Autodesk Inventor part; units mm, degrees
(part 2 of 2)
sketch "Skizze29" plane through (89.6, -2.4765, -33.8) normal (0, 0, -1) x (-1, 0, 0)
  line L0 (43.6, -0.4235) -> (43.6, -0.5235) construction
  line L1 (43.6, -0.5235) -> (49.9, -0.5235) construction
  line L2 (49.9, -0.5235) -> (52.9, 2.4765) construction
  line L3 (52.9, 2.4765) -> (79.4, 2.4765) construction
  line L4 (79.4, 2.4765) -> (79.4, 2.2765) construction
  line L5 (79.4, 2.2765) -> (83.4, 2.2765) construction
  line L6 (83.4, 2.2765) -> (83.4, 7.3765) construction
  line L7 (83.4, 7.3765) -> (49.9, 7.3765) construction
  line L8 (49.9, 7.3765) -> (49.9, 6.7966) construction
  line L9 (49.9, 6.7966) -> (45.4981, 2.3946) construction
  line L10 (45.4981, 2.3946) -> (38.1019, 2.3946) construction
  line L11 (38.1019, 2.3946) -> (33.7, 6.7966) construction
  line L12 (33.7, 6.7966) -> (33.7, 7.3765) construction
  line L13 (33.7, 7.3765) -> (17.2925, 7.3765) construction
  line L14 (17.2925, 7.3765) -> (17.2925, 2.4765) construction
  line L15 (17.2925, 2.4765) -> (31.9, 2.4765) construction
  line L16 (31.9, 2.4765) -> (34.8, -0.4235) construction
  line L17 (34.8, -0.4235) -> (43.6, -0.4235) construction
  line L18 (43.6, -28.4235) -> (34.8, -28.4235) construction
  line L19 (31.9, -31.3235) -> (34.8, -28.4235) construction
  line L20 (17.2925, -31.3235) -> (31.9, -31.3235) construction
  line L21 (17.2925, -31.3235) -> (17.2925, -36.2235) construction
  line L22 (33.7, -36.2235) -> (17.2925, -36.2235) construction
  line L23 (33.7, -36.2235) -> (33.7, -35.6437) construction
  line L24 (38.1019, -31.2417) -> (33.7, -35.6437) construction
  line L25 (45.4981, -31.2417) -> (38.1019, -31.2417) construction
  line L26 (49.9, -35.6437) -> (45.4981, -31.2417) construction
  line L27 (49.9, -35.6437) -> (49.9, -36.2235) construction
  line L28 (83.4, -36.2235) -> (49.9, -36.2235) construction
  line L29 (83.4, -31.1235) -> (83.4, -36.2235) construction
  line L30 (83.4, -31.1235) -> (79.4, -31.1235) construction
  line L31 (79.4, -31.3235) -> (79.4, -31.1235) construction
  line L32 (52.9, -31.3235) -> (79.4, -31.3235) construction
  line L33 (49.9, -28.3235) -> (52.9, -31.3235) construction
  line L34 (43.6, -28.3235) -> (49.9, -28.3235) construction
  line L35 (43.6, -28.3235) -> (43.6, -28.4235) construction
  line L36 (6, -28.8471) -> (0, -28.8471) construction
  line L37 (0, -28.8471) -> (0, -36.2235) construction
  line L38 (0, -36.2235) -> (6, -36.2235) construction
  line L39 (6, -36.2235) -> (6, -28.8471) construction
  line L40 (0, 7.3765) -> (0, 0) construction
  line L41 (0, 0) -> (6, 0) construction
  line L42 (6, 0) -> (6, 7.3765) construction
  line L43 (6, 7.3765) -> (0, 7.3765) construction
  line L44 (0, -28.8471) -> (3.8, -28.8471) construction
  line L45 (3.8, -27.1235) -> (3.8, -28.8471) construction
  line L46 (-4.5838, -27.1235) -> (3.8, -27.1235) construction
  line L47 (-4.5838, -1.7235) -> (-4.5838, -27.1235) construction
  line L48 (-4.5838, -1.7235) -> (3.8, -1.7235) construction
  line L49 (3.8, -1.7235) -> (3.8, 0) construction
  line L50 (3.8, 0) -> (0, 0) construction
  line L51 (0, 0) -> (0, 2.2765) construction
  line L52 (0, 2.2765) -> (-8.2, 2.2765) construction
  line L53 (-8.2, 2.2765) -> (-8.2, -31.1235) construction
  line L54 (0, -31.1235) -> (-8.2, -31.1235) construction
  line L55 (0, -31.1235) -> (0, -28.8471) construction
  line L56 (17.2925, 7.3765) -> (-8.2, 7.3765)
  line L57 (-8.2, 7.3765) -> (-8.2, -36.2235)
  line L58 (-8.2, -36.2235) -> (17.2925, -36.2235)
  line L59 (17.2925, -36.2235) -> (17.2925, 7.3765)
  line L60 (0, -36.2235) -> (6, -36.2235) projected
  point P0 (89.6, 2.4765)
  point P1 (3.8, 2.4765)
  constraints: 8 end point, 2 collinear, 2 parallel, 1 horizontal, 1 perpendicular
extrude "Extrusion29" cut sketch "Skizze29" against normal through all
sketch "Skizze30" plane through (0, 0, 0) normal (0, 0, 1) x (1, 0, 0)
  line L0 (72.3075, -38.7) -> (72.3075, -33.8) construction
  line L1 (57.7, -33.8) -> (72.3075, -33.8) construction
  line L2 (57.7, -33.8) -> (54.8, -30.9) construction
  line L3 (54.8, -30.9) -> (42, -30.9) construction
  line L4 (42, -30.9) -> (42, -30.8) construction
  line L5 (42, -30.8) -> (39.7, -30.8) construction
  line L6 (39.7, -30.8) -> (36.7, -33.8) construction
  line L7 (10.2, -33.8) -> (36.7, -33.8) construction
  line L8 (10.2, -29.4029) -> (10.2, -33.8) construction
  arc A0 (10.2, -4.3971) -> (10.2, -29.4029) centre (14.0958, -16.9) ccw construction
  line L9 (10.2, -4.3971) -> (10.2, 0) construction
  line L10 (10.2, 0) -> (36.7, 0) construction
  line L11 (39.7, -3) -> (36.7, 0) construction
  line L12 (42, -3) -> (39.7, -3) construction
  line L13 (42, -3) -> (42, -2.9) construction
  line L14 (42, -2.9) -> (54.8, -2.9) construction
  line L15 (57.7, 0) -> (54.8, -2.9) construction
  line L16 (57.7, 0) -> (72.3075, 0) construction
  line L17 (72.3075, 0) -> (72.3075, 4.9) construction
  line L18 (72.3075, 4.9) -> (55.9, 4.9) construction
  line L19 (55.9, 4.9) -> (55.9, 4.3201) construction
  line L20 (51.4981, -0.0818) -> (55.9, 4.3201) construction
  line L21 (44.1019, -0.0818) -> (51.4981, -0.0818) construction
  line L22 (39.7, 4.3201) -> (44.1019, -0.0818) construction
  line L23 (39.7, 4.3201) -> (39.7, 4.9) construction
  line L24 (39.7, 4.9) -> (6.2, 4.9) construction
  line L25 (6.2, 4.9) -> (6.2, -0.2) construction
  line L26 (6.2, -0.2) -> (-2, -0.2) construction
  line L27 (-2, -0.2) -> (-2, -33.6) construction
  line L28 (6.2, -33.6) -> (-2, -33.6) construction
  line L29 (6.2, -38.7) -> (6.2, -33.6) construction
  line L30 (39.7, -38.7) -> (6.2, -38.7) construction
  line L31 (39.7, -38.7) -> (39.7, -38.1201) construction
  line L32 (39.7, -38.1201) -> (44.1019, -33.7182) construction
  line L33 (44.1019, -33.7182) -> (51.4981, -33.7182) construction
  line L34 (51.4981, -33.7182) -> (55.9, -38.1201) construction
  line L35 (55.9, -38.1201) -> (55.9, -38.7) construction
  line L36 (72.3075, -38.7) -> (55.9, -38.7) construction
  circle A1 centre (59.1, -36.25) radius 1.4
  line L37 (-16.8615, -16.9) -> (87.169, -16.9) construction
  circle A2 centre (59.1, 2.45) radius 1.4
  line L38 (72.3075, -38.7) -> (72.3075, -33.8) construction
  line L39 (72.3075, -36.25) -> (54.0299, -36.25) construction
  line L40 (51.4981, -33.7182) -> (55.9, -38.1201) construction
  line L41 (57.7, -33.8) -> (54.8, -30.9) construction
  line L42 (57.7, -33.8) -> (57.7, -38.7) construction
  point P0 (0, 0)
  dimension "d149" = 2.8
  constraints: 4 end point, 3 point on line, 2 centre point, 1 horizontal, 1 midpoint, 1 symmetric about line, 1 tangent, 1 vertical, 1 other
  measures "d149" diameter of A1
extrude "Extrusion30" cut sketch "Skizze30" against normal through all
fillet "Rundung1" radius 3 2 edges at (72.3075, -38.7, -3) (72.3075, 4.9, -3)
sketch "Skizze31" plane through (0, 0, 0) normal (0, 0, 1) x (1, 0, 0)
  circle A0 centre (59.1, -36.25) radius 1.4 construction
  circle A1 centre (59.1, 2.45) radius 1.4 construction
  arc A2 (72.3075, 1.9) -> (69.3075, 4.9) centre (69.3075, 1.9) ccw construction
  line L0 (69.3075, 4.9) -> (55.9, 4.9) construction
  line L1 (55.9, 4.9) -> (55.9, 4.3201) construction
  line L2 (51.4981, -0.0818) -> (55.9, 4.3201) construction
  line L3 (44.1019, -0.0818) -> (51.4981, -0.0818) construction
  line L4 (39.7, 4.3201) -> (44.1019, -0.0818) construction
  line L5 (39.7, 4.3201) -> (39.7, 4.9) construction
  line L6 (39.7, 4.9) -> (6.2, 4.9) construction
  line L7 (6.2, 4.9) -> (6.2, -0.2) construction
  line L8 (6.2, -0.2) -> (-2, -0.2) construction
  line L9 (-2, -0.2) -> (-2, -33.6) construction
  line L10 (6.2, -33.6) -> (-2, -33.6) construction
  line L11 (6.2, -38.7) -> (6.2, -33.6) construction
  line L12 (39.7, -38.7) -> (6.2, -38.7) construction
  line L13 (39.7, -38.7) -> (39.7, -38.1201) construction
  line L14 (39.7, -38.1201) -> (44.1019, -33.7182) construction
  line L15 (44.1019, -33.7182) -> (51.4981, -33.7182) construction
  line L16 (51.4981, -33.7182) -> (55.9, -38.1201) construction
  line L17 (55.9, -38.1201) -> (55.9, -38.7) construction
  line L18 (69.3075, -38.7) -> (55.9, -38.7) construction
  arc A3 (69.3075, -38.7) -> (72.3075, -35.7) centre (69.3075, -35.7) ccw construction
  line L19 (72.3075, -35.7) -> (72.3075, -33.8) construction
  line L20 (57.7, -33.8) -> (72.3075, -33.8) construction
  line L21 (57.7, -33.8) -> (54.8, -30.9) construction
  line L22 (54.8, -30.9) -> (42, -30.9) construction
  line L23 (42, -30.9) -> (42, -30.8) construction
  line L24 (42, -30.8) -> (39.7, -30.8) construction
  line L25 (39.7, -30.8) -> (36.7, -33.8) construction
  line L26 (10.2, -33.8) -> (36.7, -33.8) construction
  line L27 (10.2, -29.4029) -> (10.2, -33.8) construction
  arc A4 (10.2, -4.3971) -> (10.2, -29.4029) centre (14.0958, -16.9) ccw construction
  line L28 (10.2, -4.3971) -> (10.2, 0) construction
  line L29 (10.2, 0) -> (36.7, 0) construction
  line L30 (39.7, -3) -> (36.7, 0) construction
  line L31 (42, -3) -> (39.7, -3) construction
  line L32 (42, -3) -> (42, -2.9) construction
  line L33 (42, -2.9) -> (54.8, -2.9) construction
  line L34 (57.7, 0) -> (54.8, -2.9) construction
  line L35 (57.7, 0) -> (72.3075, 0) construction
  line L36 (72.3075, 0) -> (72.3075, 1.9) construction
  line L37 (6.2, 4.9) -> (39.8, 4.9)
  line L38 (39.8, 4.9) -> (39.8, 8)
  line L39 (39.8, 8) -> (6.2, 8)
  line L40 (6.2, 8) -> (6.2, 4.9)
  line L41 (-16.9858, -16.9) -> (87.9146, -16.9) projected
  line L42 (39.7, -38.1201) -> (39.7, -38.7) construction
  line L43 (39.7, -38.7) -> (6.2, -38.7) construction
  line L44 (6.2, -38.7) -> (39.8, -38.7)
  line L45 (39.8, -38.7) -> (39.8, -41.8)
  line L46 (39.8, -41.8) -> (6.2, -41.8)
  line L47 (6.2, -41.8) -> (6.2, -38.7)
  point P0 (0, 0)
  dimension "d153" = 33.6
  dimension "d154" = 49.8
  constraints: 20 end point, 3 symmetric about line, 2 parallel, 1 horizontal, 1 perpendicular
  measures "d153" distance of L38.end L39.end
  measures "d154" distance between parallel lines of L46 L39
extrude "Extrusion31" add sketch "Skizze31" against normal up to surface (6 mm away)
sketch "Sketch32" plane through (0, 0, -6) normal (0, 0, -1) x (-1, 0, 0)
  circle A0 centre (-59.1, -36.25) radius 1.4 projected
  circle A1 centre (-59.1, 2.45) radius 1.4 projected
  arc A2 (-69.3075, 4.9) -> (-72.3075, 1.9) centre (-69.3075, 1.9) ccw projected
  line L0 (-69.3075, 4.9) -> (-55.9, 4.9) projected
  line L1 (-55.9, 4.9) -> (-55.9, 4.3201) projected
  line L2 (-51.4981, -0.0818) -> (-55.9, 4.3201) projected
  line L3 (-44.1019, -0.0818) -> (-51.4981, -0.0818) projected
  line L4 (-39.7, 4.3201) -> (-44.1019, -0.0818) projected
  line L5 (-39.7, 4.3201) -> (-39.7, 4.9) projected
  line L6 (-39.7, 4.9) -> (-39.8, 4.9) projected
  line L7 (-39.8, 4.9) -> (-39.8, 8) projected
  line L8 (-39.8, 8) -> (-6.2, 8) projected
  line L9 (-6.2, 8) -> (-6.2, -0.2) projected
  line L10 (-6.2, -0.2) -> (2, -0.2) projected
  line L11 (2, -0.2) -> (2, -33.6) projected
  line L12 (-6.2, -33.6) -> (2, -33.6) projected
  line L13 (-6.2, -41.8) -> (-6.2, -33.6) projected
  line L14 (-39.8, -41.8) -> (-6.2, -41.8) projected
  line L15 (-39.8, -38.7) -> (-39.8, -41.8) projected
  line L16 (-39.7, -38.7) -> (-39.8, -38.7) projected
  line L17 (-39.7, -38.7) -> (-39.7, -38.1201) projected
  line L18 (-39.7, -38.1201) -> (-44.1019, -33.7182) projected
  line L19 (-44.1019, -33.7182) -> (-51.4981, -33.7182) projected
  line L20 (-51.4981, -33.7182) -> (-55.9, -38.1201) projected
  line L21 (-55.9, -38.1201) -> (-55.9, -38.7) projected
  line L22 (-69.3075, -38.7) -> (-55.9, -38.7) projected
  arc A3 (-72.3075, -35.7) -> (-69.3075, -38.7) centre (-69.3075, -35.7) ccw projected
  line L23 (-72.3075, -35.7) -> (-72.3075, -33.8) projected
  line L24 (-57.7, -33.8) -> (-72.3075, -33.8) projected
  line L25 (-57.7, -33.8) -> (-54.8, -30.9) projected
  line L26 (-54.8, -30.9) -> (-42, -30.9) projected
  line L27 (-42, -30.9) -> (-42, -30.8) projected
  line L28 (-42, -30.8) -> (-39.7, -30.8) projected
  line L29 (-39.7, -30.8) -> (-36.7, -33.8) projected
  line L30 (-10.2, -33.8) -> (-36.7, -33.8) projected
  line L31 (-10.2, -29.4029) -> (-10.2, -33.8) projected
  arc A4 (-10.2, -29.4029) -> (-10.2, -4.3971) centre (-14.0958, -16.9) ccw projected
  line L32 (-10.2, -4.3971) -> (-10.2, 0) projected
  line L33 (-10.2, 0) -> (-36.7, 0) projected
  line L34 (-39.7, -3) -> (-36.7, 0) projected
  line L35 (-42, -3) -> (-39.7, -3) projected
  line L36 (-42, -3) -> (-42, -2.9) projected
  line L37 (-42, -2.9) -> (-54.8, -2.9) projected
  line L38 (-57.7, 0) -> (-54.8, -2.9) projected
  line L39 (-57.7, 0) -> (-72.3075, 0) projected
  line L40 (-72.3075, 0) -> (-72.3075, 1.9) projected
  line L41 (-48.0005, -33.7182) -> (-48.0005, -30.9)
  line L42 (-54.8, -30.9) -> (-42, -30.9) projected
  line L43 (-54.8, -2.9) -> (-46, -2.9) projected
  line L44 (-48.0005, -2.9) -> (-48.0005, -0.0818)
  line L45 (-44.1019, -0.0818) -> (-51.4981, -0.0818) projected
  point P0 (0, 0)
  dimension "d157" = 24.307
  constraints: 6 point on line, 4 end point, 1 perpendicular
  measures "d157" distance between parallel lines of L23 L41
extrude "Extrusion32" add sketch "Sketch32" along normal blind 7 contours A0 | A1 | L0 L1 L2 L3 L44 L37 L38 L39 L40 A2 | L41 L19 L20 L21 L22 A3 L23 L24 L25 L26
sketch "Sketch33" plane through (0, 0, 0) normal (0, 0, 1) x (1, 0, 0)
  circle A0 centre (59.1, -36.25) radius 1.4 projected
  circle A1 centre (59.1, 2.45) radius 1.4 projected
  arc A2 (72.3075, 1.9) -> (69.3075, 4.9) centre (69.3075, 1.9) ccw projected
  line L0 (69.3075, 4.9) -> (55.9, 4.9) projected
  line L1 (55.9, 4.9) -> (55.9, 4.3201) projected
  line L2 (51.4981, -0.0818) -> (55.9, 4.3201) projected
  line L3 (44.1019, -0.0818) -> (51.4981, -0.0818) projected
  line L4 (39.7, 4.3201) -> (44.1019, -0.0818) projected
  line L5 (39.7, 4.3201) -> (39.7, 4.9) projected
  line L6 (39.7, 4.9) -> (39.8, 4.9) projected
  line L7 (39.8, 4.9) -> (39.8, 8) projected
  line L8 (39.8, 8) -> (6.2, 8) projected
  line L9 (6.2, 8) -> (6.2, -0.2) projected
  line L10 (6.2, -0.2) -> (-2, -0.2) projected
  line L11 (-2, -0.2) -> (-2, -33.6) projected
  line L12 (6.2, -33.6) -> (-2, -33.6) projected
  line L13 (6.2, -41.8) -> (6.2, -33.6) projected
  line L14 (39.8, -41.8) -> (6.2, -41.8) projected
  line L15 (39.8, -38.7) -> (39.8, -41.8) projected
  line L16 (39.7, -38.7) -> (39.8, -38.7) projected
  line L17 (39.7, -38.7) -> (39.7, -38.1201) projected
  line L18 (39.7, -38.1201) -> (44.1019, -33.7182) projected
  line L19 (44.1019, -33.7182) -> (51.4981, -33.7182) projected
  line L20 (51.4981, -33.7182) -> (55.9, -38.1201) projected
  line L21 (55.9, -38.1201) -> (55.9, -38.7) projected
  line L22 (69.3075, -38.7) -> (55.9, -38.7) projected
  arc A3 (69.3075, -38.7) -> (72.3075, -35.7) centre (69.3075, -35.7) ccw projected
  line L23 (72.3075, -35.7) -> (72.3075, -33.8) projected
  line L24 (57.7, -33.8) -> (72.3075, -33.8) projected
  line L25 (57.7, -33.8) -> (54.8, -30.9) projected
  line L26 (54.8, -30.9) -> (42, -30.9) projected
  line L27 (42, -30.9) -> (42, -30.8) projected
  line L28 (42, -30.8) -> (39.7, -30.8) projected
  line L29 (39.7, -30.8) -> (36.7, -33.8) projected
  line L30 (10.2, -33.8) -> (36.7, -33.8) projected
  line L31 (10.2, -29.4029) -> (10.2, -33.8) projected
  arc A4 (10.2, -4.3971) -> (10.2, -29.4029) centre (14.0958, -16.9) ccw projected
  line L32 (10.2, -4.3971) -> (10.2, 0) projected
  line L33 (10.2, 0) -> (36.7, 0) projected
  line L34 (39.7, -3) -> (36.7, 0) projected
  line L35 (42, -3) -> (39.7, -3) projected
  line L36 (42, -3) -> (42, -2.9) projected
  line L37 (42, -2.9) -> (54.8, -2.9) projected
  line L38 (57.7, 0) -> (54.8, -2.9) projected
  line L39 (57.7, 0) -> (72.3075, 0) projected
  line L40 (72.3075, 0) -> (72.3075, 1.9) projected
  line L41 (69.3075, 4.9) -> (55.9, 4.9) projected
  line L42 (55.9, 4.9) -> (48.0005, 4.9)
  line L43 (48.0005, 4.9) -> (48.0005, -0.0818)
  line L44 (44.1019, -33.7182) -> (51.4981, -33.7182) projected
  line L45 (48.0005, -33.7182) -> (48.0005, -38.7)
  line L46 (48.0005, -38.7) -> (55.9, -38.7)
  point P0 (0, 0)
  dimension "d160" = 24.307
  constraints: 8 end point, 4 point on line, 2 perpendicular, 1 horizontal
  measures "d160" distance between parallel lines of L40 L43
extrude "Extrusion33" add sketch "Sketch33" against normal up to surface (13 mm away) contours A0 | A1 | L1 L2 L3 L43 L42 | L19 L20 L21 L46 L45
sketch "Sketch34" plane through (0, 0, -13) normal (0, 0, -1) x (-1, 0, 0)
  line L0 (-48.0005, -38.7) -> (-48.0005, -30.9) projected
  line L1 (-48.0005, -30.9) -> (-54.8, -30.9) projected
  line L2 (-54.8, -30.9) -> (-57.7, -33.8) projected
  line L3 (-57.7, -33.8) -> (-72.3075, -33.8) projected
  line L4 (-72.3075, -33.8) -> (-72.3075, -35.7) projected
  arc A0 (-72.3075, -35.7) -> (-69.3075, -38.7) centre (-69.3075, -35.7) ccw projected
  line L5 (-69.3075, -38.7) -> (-48.0005, -38.7) projected
  line L6 (-72.3075, 1.9) -> (-72.3075, 0) projected
  line L7 (-72.3075, 0) -> (-57.7, 0) projected
  line L8 (-57.7, 0) -> (-54.8, -2.9) projected
  line L9 (-54.8, -2.9) -> (-48.0005, -2.9) projected
  line L10 (-48.0005, -2.9) -> (-48.0005, 4.9) projected
  line L11 (-48.0005, 4.9) -> (-69.3075, 4.9) projected
  arc A1 (-69.3075, 4.9) -> (-72.3075, 1.9) centre (-69.3075, 1.9) ccw projected
  line L12 (-48.0005, -0.0818) -> (-48.0005, -2.9) projected
  line L13 (-48.0005, -30.9) -> (-48.0005, -2.9)
  line L14 (-72.3075, -33.8) -> (-72.3075, 0)
  point P0 (0, 0)
  constraints: 4 end point, 2 vertical
extrude "Extrusion34" add sketch "Sketch34" along normal blind 1
sketch "Sketch35" plane through (0, 0, -14) normal (0, 0, -1) x (-1, 0, 0)
  line L0 (-48.0005, -38.7) -> (-48.0005, 4.9) projected
  line L1 (-48.0005, 4.9) -> (-69.3075, 4.9) projected
  arc A0 (-69.3075, 4.9) -> (-72.3075, 1.9) centre (-69.3075, 1.9) ccw projected
  line L2 (-72.3075, 1.9) -> (-72.3075, -35.7) projected
  arc A1 (-72.3075, -35.7) -> (-69.3075, -38.7) centre (-69.3075, -35.7) ccw projected
  line L3 (-69.3075, -38.7) -> (-48.0005, -38.7) projected
  line L4 (-87.9146, -16.9) -> (16.9858, -16.9) construction
  line L5 (-48.0005, -33.8) -> (-72.3075, -33.8)
  line L6 (-72.3075, 1.9) -> (-72.3075, -35.7) construction
  line L7 (-48.0005, 0) -> (-72.3075, 0)
  line L8 (-48.0005, -33.7182) -> (-48.0005, -38.7) projected
  line L9 (-48.0005, -33.8) -> (-48.0005, -38.7)
  line L10 (-48.0005, -38.7) -> (-69.3075, -38.7)
  arc A2 (-72.3075, -35.7) -> (-69.3075, -38.7) centre (-69.3075, -35.7) ccw projected
  line L11 (-72.3075, -33.8) -> (-72.3075, -35.7)
  line L12 (-48.0005, 4.9) -> (-48.0005, -0.0818) projected
  line L13 (-48.0005, 0) -> (-48.0005, 4.9)
  line L14 (-48.0005, 4.9) -> (-69.3075, 4.9)
  line L15 (-69.263, 4.9) -> (-66.363, 4.9) projected
  line L16 (-72.3075, 0) -> (-72.3075, 1.9) projected
  line L17 (-72.3075, 0) -> (-72.3075, 1.9)
  arc A3 (-69.3075, 4.9) -> (-72.3075, 1.9) centre (-69.3075, 1.9) ccw projected
  arc A4 (-69.3075, 4.9) -> (-72.3075, 1.9) centre (-69.3075, 1.9) ccw
  arc A5 (-72.3075, -35.7) -> (-69.3075, -38.7) centre (-69.3075, -35.7) ccw
  point P0 (0, 0)
  dimension "d165" = 4.9
  constraints: 16 end point, 4 collinear, 4 point on circle, 2 centre point, 2 concentric, 2 perpendicular, 2 point on line, 2 symmetric about line, 2 tangent, 1 vertical
  measures "d165" distance between parallel lines of L3 L5
extrude "Extrusion35" add sketch "Sketch35" along normal blind 5.5 contours L3 A1 L2 L5 L0 | L2 A0 L1 L0 L7
sketch "Sketch36" plane through (0, 0, -19.5) normal (0, 0, -1) x (-1, 0, 0)
  line L0 (-48.0005, -38.7) -> (-48.0005, -33.8) projected
  line L1 (-48.0005, -33.8) -> (-72.3075, -33.8) projected
  line L2 (-72.3075, -33.8) -> (-72.3075, -35.7) projected
  arc A0 (-72.3075, -35.7) -> (-69.3075, -38.7) centre (-69.3075, -35.7) ccw projected
  line L3 (-69.3075, -38.7) -> (-48.0005, -38.7) projected
  line L4 (-72.3075, -33.8) -> (-48.0005, -33.8) projected
  line L5 (-48.0005, -33.8) -> (-48.0005, 0) projected
  line L6 (-48.0005, 0) -> (-72.3075, 0) projected
  line L7 (-72.3075, 0) -> (-72.3075, -33.8) projected
  line L8 (-48.0005, 4.9) -> (-69.3075, 4.9) projected
  arc A1 (-69.3075, 4.9) -> (-72.3075, 1.9) centre (-69.3075, 1.9) ccw projected
  line L9 (-72.3075, 1.9) -> (-72.3075, 0) projected
  line L10 (-72.3075, 0) -> (-48.0005, 0) projected
  line L11 (-48.0005, 0) -> (-48.0005, 4.9) projected
  point P0 (0, 0)
extrude "Extrusion36" add sketch "Sketch36" along normal blind 2
sketch "Sketch37" plane through (0, 0, -21.5) normal (0, 0, -1) x (-1, 0, 0)
  line L0 (-61, -23.9) -> (-71, -23.9) construction
  line L1 (-48.0005, -38.7) -> (-48.0005, 4.9) construction
  line L2 (-48.0005, 4.9) -> (-69.3075, 4.9) construction
  arc A0 (-69.3075, 4.9) -> (-72.3075, 1.9) centre (-69.3075, 1.9) ccw construction
  line L3 (-72.3075, 1.9) -> (-72.3075, -35.7) construction
  arc A1 (-72.3075, -35.7) -> (-69.3075, -38.7) centre (-69.3075, -35.7) ccw construction
  line L4 (-69.3075, -38.7) -> (-48.0005, -38.7) construction
  line L5 (-87.9146, -16.9) -> (16.9858, -16.9) construction
  circle A2 centre (-67.2465, -16.9) radius 1.7
  point P0 (0, 0)
  dimension "d170" = 5.061
  dimension "d171" = 3.4
  constraints: 1 centre point, 1 point on line
  measures "d170" distance from line of L3 A2.centre
  measures "d171" diameter of A2
extrude "Extrusion37" cut sketch "Sketch37" against normal up to surface (8.5 mm away)
sketch "Sketch38" plane through (0, 0, -13) normal (0, 0, 1) x (1, 0, 0)
  circle A0 centre (67.2465, -16.9) radius 1.7 construction
  line L0 (54.8, -2.9) -> (48.0005, -2.9) construction
  line L1 (48.0005, -30.9) -> (48.0005, -2.9) construction
  line L2 (48.0005, -30.9) -> (54.8, -30.9) construction
  line L3 (54.8, -30.9) -> (57.7, -33.8) construction
  line L4 (57.7, -33.8) -> (72.3075, -33.8) construction
  line L5 (72.3075, 0) -> (72.3075, -33.8) construction
  line L6 (72.3075, 0) -> (57.7, 0) construction
  line L7 (57.7, 0) -> (54.8, -2.9) construction
  circle A1 centre (67.2465, -16.9) radius 2.3
  point P0 (0, 0)
  dimension "d174" = 0.6
  constraints: 1 centre point
  measures "d174" radial gap between concentric circles of A0 A1
extrude "Extrusion38" cut sketch "Sketch38" against normal up to surface (1 mm away)
sketch "Sketch39" plane through (0, 0, -21.5) normal (0, 0, -1) x (-1, 0, 0)
  circle A0 centre (-67.2465, -16.9) radius 1.7 construction
  line L0 (-48.0005, -38.7) -> (-48.0005, 4.9) construction
  line L1 (-48.0005, 4.9) -> (-69.3075, 4.9) construction
  arc A1 (-69.3075, 4.9) -> (-72.3075, 1.9) centre (-69.3075, 1.9) ccw construction
  line L2 (-72.3075, 1.9) -> (-72.3075, -35.7) construction
  arc A2 (-72.3075, -35.7) -> (-69.3075, -38.7) centre (-69.3075, -35.7) ccw construction
  line L3 (-69.3075, -38.7) -> (-48.0005, -38.7) construction
  line L4 (-49.7605, -33.742) -> (-54.8216, -33.742) construction
  line L5 (-54.8216, -33.742) -> (-54.8216, -27.0483) construction
  line L6 (-54.8216, -27.0483) -> (-49.7605, -27.0483) construction
  line L7 (-49.7605, -27.0483) -> (-49.7605, -33.742) construction
  line L8 (-49.7605, -4.0192) -> (-54.9849, -4.0192) construction
  line L9 (-54.9849, -4.0192) -> (-54.9849, 2.6745) construction
  line L10 (-54.9849, 2.6745) -> (-49.7605, 2.6745) construction
  line L11 (-49.7605, 2.6745) -> (-49.7605, -4.0192) construction
  line L12 (-50.1879, -33.6727) -> (-52.0242, -33.6727)
  spline S0 degree 2 poles (-52.0242, -33.6727) (-52.5671, -33.6727) (-53.2369, -33.3763) (-53.672, -32.8258) (-53.8683, -32.0943) (-53.8683, -31.6862) knots 0 0 0 1 2 3 4 4 4
  spline S1 degree 2 poles (-53.8683, -31.6862) (-53.8683, -31.0433) (-53.5757, -30.3388) (-53.0598, -29.8614) (-52.7596, -29.7805) knots 0 0 0 1 2 3 3 3
  spline S2 degree 2 poles (-52.7596, -29.7805) (-52.3553, -29.6727) (-52.0242, -29.6727) knots 0 0 0 1 1 1
  line L13 (-52.0242, -29.6727) -> (-50.1879, -29.6727)
  line L14 (-50.1879, -29.6727) -> (-50.1879, -33.6727)
  line L15 (-51.4237, -32.768) -> (-51.4237, -30.5813)
  line L16 (-51.4237, -30.5813) -> (-51.7278, -30.5813)
  spline S3 degree 2 poles (-51.7278, -30.5813) (-52.1128, -30.5813) (-52.44, -30.7545) (-52.6248, -31.1819) (-52.6248, -31.6631) knots 0 0 0 1 2 3 3 3
  spline S4 degree 2 poles (-52.6248, -31.6631) (-52.6248, -32.2983) (-52.209, -32.768) (-51.7316, -32.768) knots 0 0 0 1 2 2 2
  line L17 (-51.7316, -32.768) -> (-51.4237, -32.768)
  spline S5 degree 2 poles (-54.3649, -31.6708) (-54.3649, -32.6487) (-55.4583, -33.742) (-56.4323, -33.742) knots 0 0 0 1 2 2 2
  spline S6 degree 2 poles (-56.4323, -33.742) (-57.4294, -33.742) (-58.5112, -32.6679) (-58.5112, -31.7016) knots 0 0 0 1 2 2 2
  spline S7 degree 2 poles (-58.5112, -31.7016) (-58.5112, -31.0009) (-58.0377, -30.1039) (-57.1445, -29.6034) (-56.4785, -29.6034) knots 0 0 0 1 2 3 3 3
  spline S8 degree 2 poles (-56.4785, -29.6034) (-55.8048, -29.6034) (-54.9155, -30.0346) (-54.3649, -30.9701) (-54.3649, -31.6708) knots 0 0 0 1 2 3 3 3
  spline S9 degree 2 poles (-55.6008, -31.6631) (-55.6008, -31.0587) (-56.0512, -30.5274) (-56.44, -30.5274) knots 0 0 0 1 2 2 2
  spline S10 degree 2 poles (-56.44, -30.5274) (-56.8366, -30.5274) (-57.2754, -31.0471) (-57.2754, -31.717) knots 0 0 0 1 2 2 2
  spline S11 degree 2 poles (-57.2754, -31.717) (-57.2754, -32.2829) (-56.8212, -32.8065) (-56.4285, -32.8065) knots 0 0 0 1 2 2 2
  spline S12 degree 2 poles (-56.4285, -32.8065) (-56.055, -32.8065) (-55.6008, -32.2752) (-55.6008, -31.6631) knots 0 0 0 1 2 2 2
  line L18 (-58.7653, -33.6727) -> (-59.9395, -33.6727)
  line L19 (-59.9395, -33.6727) -> (-60.363, -31.436)
  line L20 (-60.363, -31.436) -> (-60.9828, -33.6727)
  line L21 (-60.9828, -33.6727) -> (-62.1494, -33.6727)
  line L22 (-62.1494, -33.6727) -> (-62.7692, -31.4437)
  line L23 (-62.7692, -31.4437) -> (-63.1965, -33.6727)
  line L24 (-63.1965, -33.6727) -> (-64.363, -33.6727)
  line L25 (-64.363, -33.6727) -> (-63.4814, -29.6727)
  line L26 (-63.4814, -29.6727) -> (-62.2687, -29.6727)
  line L27 (-62.2687, -29.6727) -> (-61.568, -32.1905)
  line L28 (-61.568, -32.1905) -> (-60.8674, -29.6727)
  line L29 (-60.8674, -29.6727) -> (-59.6546, -29.6727)
  line L30 (-59.6546, -29.6727) -> (-58.7653, -33.6727)
  line L31 (-64.775, -33.6727) -> (-65.9299, -33.6727)
  line L32 (-65.9299, -33.6727) -> (-67.4391, -31.4591)
  line L33 (-67.4391, -31.4591) -> (-67.4391, -33.6727)
  line L34 (-67.4391, -33.6727) -> (-68.6056, -33.6727)
  line L35 (-68.6056, -33.6727) -> (-68.6056, -29.6727)
  line L36 (-68.6056, -29.6727) -> (-67.4391, -29.6727)
  line L37 (-67.4391, -29.6727) -> (-65.9376, -31.8748)
  line L38 (-65.9376, -31.8748) -> (-65.9376, -29.6727)
  line L39 (-65.9376, -29.6727) -> (-64.775, -29.6727)
  line L40 (-64.775, -29.6727) -> (-64.775, -33.6727)
  line L41 (-52.7788, -4.0192) -> (-54.0108, -4.0192)
  line L42 (-54.0108, -4.0192) -> (-54.0108, -1.6361)
  spline S13 degree 2 poles (-54.0108, -1.6361) (-54.0108, -1.2819) (-53.7913, -0.6505) (-53.3178, -0.1809) (-53.056, -0.0846) knots 0 0 0 1 2 3 3 3
  spline S14 degree 2 poles (-53.056, -0.0846) (-52.698, 0.0501) (-52.1898, 0.0501) knots 0 0 0 1 1 1
  spline S15 degree 2 poles (-52.1898, 0.0501) (-51.8972, 0.0501) (-51.2081, -0.0307) (-50.7422, -0.2733) (-50.3572, -0.7198) (-50.2879, -0.9585) knots 0 0 0 1 2 3 4 4 4
  spline S16 degree 2 poles (-50.2879, -0.9585) (-50.1725, -1.3397) (-50.1725, -1.6361) knots 0 0 0 1 1 1
  line L43 (-50.1725, -1.6361) -> (-50.1725, -4.0192)
  line L44 (-50.1725, -4.0192) -> (-51.4044, -4.0192)
  line L45 (-51.4044, -4.0192) -> (-51.4044, -1.5784)
  spline S17 degree 2 poles (-51.4044, -1.5784) (-51.4044, -1.2511) (-51.7701, -0.8815) (-52.0935, -0.8815) knots 0 0 0 1 2 2 2
  spline S18 degree 2 poles (-52.0935, -0.8815) (-52.4131, -0.8815) (-52.7788, -1.2434) (-52.7788, -1.5784) knots 0 0 0 1 2 2 2
  line L46 (-52.7788, -1.5784) -> (-52.7788, -4.0192)
  line L47 (-54.8231, -4.0192) -> (-56.8789, -4.0192)
  spline S19 degree 2 poles (-56.8789, -4.0192) (-57.5488, -4.0192) (-58.2187, -3.3801) (-58.2187, -2.7911) knots 0 0 0 1 2 2 2
  spline S20 degree 2 poles (-58.2187, -2.7911) (-58.2187, -2.1828) (-57.491, -1.5014) (-56.7442, -1.5014) knots 0 0 0 1 2 2 2
  line L48 (-56.7442, -1.5014) -> (-56.0666, -1.5014)
  line L49 (-56.0666, -1.5014) -> (-56.0666, -0.0192)
  line L50 (-56.0666, -0.0192) -> (-54.8231, -0.0192)
  line L51 (-54.8231, -0.0192) -> (-54.8231, -4.0192)
  line L52 (-56.0666, -2.3137) -> (-56.3669, -2.3137)
  spline S21 degree 2 poles (-56.3669, -2.3137) (-56.7249, -2.3137) (-57.0136, -2.5639) (-57.0136, -2.7564) knots 0 0 0 1 2 2 2
  spline S22 degree 2 poles (-57.0136, -2.7564) (-57.0136, -2.9451) (-56.7634, -3.2069) (-56.4169, -3.2069) knots 0 0 0 1 2 2 2
  line L53 (-56.4169, -3.2069) -> (-56.0666, -3.2069)
  line L54 (-56.0666, -3.2069) -> (-56.0666, -2.3137)
  point P0 (0, 0)
  constraints: 1 collinear, 4 other
emboss "Emboss1" sketch "Sketch39" operation cut depth 1 direction (0, 0, 1)
ref_plane "Work Plane5" through (6, -38.3, -33.8) normal (0, 0, -1) x (1, 0, 0)
ref_plane "Work Plane6" through (10.2, -29.4, -20.3) normal (0, 0, 1) x (-1, 0, 0)
ref_plane "Work Plane7" through (0, -33.8, -18) normal (0, 0, 1) x (-1, 0, 0)
body "Solid1"
